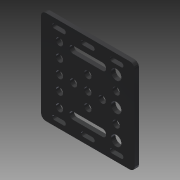
# Autodesk Inventor part: 20mm gantry plate
Saved by Autodesk Inventor 2014 SP1 (Build 180222100, 222)
## iProperties
Created: 2016-04-10
Part Number: 20mm gantry plate
Material: Generic
Document SubType Name: Modeling
Designer: Ben
Density: 1 g/cm^3
Appearance: Default
Author: Ben
Autodesk Inventor part; units mm, degrees
ref_plane "YZ Plane" through (0, 0, 0) normal (1, 0, 0) x (0, 1, 0)
ref_plane "XZ Plane" through (0, 0, 0) normal (0, 1, 0) x (-1, 0, 0)
ref_plane "XY Plane" through (0, 0, 0) normal (0, 0, 1) x (1, 0, 0)
sketch "Sketch1" plane through (0, 0, 0) normal (0, 0, 1) x (1, 0, 0)
  line L0 (-32.75, 32.75) -> (32.75, 32.75)
  line L1 (32.75, 32.75) -> (32.75, -32.75)
  line L2 (32.75, -32.75) -> (-32.75, -32.75)
  line L3 (-32.75, -32.75) -> (-32.75, 32.75)
  line L4 (0, 32.75) -> (0, -32.75) construction
  line L5 (-32.75, 0) -> (32.75, 0) construction
  point P0 (0, 0)
  dimension "d0" = 65.5
  dimension "d1" = 65.5
  constraints: 12 end point, 6 midpoint, 2 parallel, 1 horizontal, 1 perpendicular
  measures "d0" distance of L1.end L2.end
  measures "d1" distance of L0.end L1.end
extrude "Extrusion1" add sketch "Sketch1" along normal blind 3
sketch "Sketch2" plane through (0, 0, 3) normal (0, 0, 1) x (1, 0, 0)
  line L0 (32.75, 32.75) -> (-32.75, 32.75) projected
  line L1 (-32.75, 32.75) -> (-32.75, -32.75) projected
  line L2 (-32.75, -32.75) -> (32.75, -32.75) projected
  line L3 (32.75, -32.75) -> (32.75, 32.75) projected
  circle A0 centre (0, 0) radius 2.5
  circle A1 centre (0, 10) radius 2.5
  line L4 (0, 0) -> (0, 20.5611) construction
  circle A2 centre (-10, 0) radius 2.5
  circle A3 centre (0, -10) radius 2.5
  circle A4 centre (10, 0) radius 2.5
  circle A5 centre (-19.85, 0) radius 2.5
  circle A6 centre (-19.85, -10) radius 2.5
  circle A7 centre (-19.85, -20) radius 2.5
  circle A8 centre (-19.85, 10) radius 2.5
  circle A9 centre (-19.85, 0) radius 2.5
  circle A10 centre (-19.85, -10) radius 2.5
  circle A11 centre (-19.85, 20) radius 2.5
  circle A12 centre (-19.85, 10) radius 2.5
  circle A13 centre (-19.85, 0) radius 2.5
  line L5 (19.85, 32.75) -> (19.85, -32.75) construction
  circle A14 centre (19.85, 10) radius 2.5
  circle A15 centre (19.85, -10) radius 2.5
  line L6 (0, 0) -> (-32.75, 0) construction
  circle A16 centre (19.85, 0) radius 3.6
  circle A17 centre (19.85, 20) radius 3.6
  circle A18 centre (19.85, -20) radius 3.6
  circle A19 centre (19.85, 0) radius 3.6
  dimension "d4" = 5
  dimension "d5" = 5
  dimension "d6" = 10
  dimension "d9" = 360
  dimension "d11" = 5
  dimension "d12" = 12.9
  dimension "d15" = 10
  dimension "d18" = 10
  dimension "d21" = 5
  dimension "d22" = 5
  dimension "d23" = 12.9
  dimension "d24" = 10
  dimension "d25" = 7.2
  dimension "d28" = 20
  dimension "d31" = 20
  constraints: 20 centre point, 6 end point, 6 point on line, 4 vertical, 2 midpoint, 1 coincident, 1 parallel, 1 perpendicular, 1 symmetric about line, 31 other
  measures "d4" diameter of A0
  measures "d5" diameter of A1
  measures "d6" distance of L4.start A1.centre
  measures "d11" diameter of A5
  measures "d12" distance from line of A5.centre L1
  measures "d15" distance of A5.centre A6.centre
  measures "d18" distance of A5.centre A8.centre
  measures "d21" diameter of A14
  measures "d22" diameter of A15
  measures "d23" distance between parallel lines of L3 L5
  measures "d24" vertical distance of point (0, 0) A14.centre
  measures "d25" diameter of A16
  measures "d28" distance of A16.centre A17.centre
  measures "d31" distance of A16.centre A18.centre
extrude "Extrusion2" cut sketch "Sketch2" against normal up to next contours A0 | A1 | A2 | A3 | A4 | A5 | A6 | A7 | A8 | A11 | A14 | A15 | A16 | A17 | A18
sketch "Sketch3" plane through (0, 0, 3) normal (0, 0, 1) x (1, 0, 0)
  circle A0 centre (-19.85, -20) radius 2.5 projected
  circle A1 centre (0, 0) radius 2.5 projected
  line L0 (32.75, 32.75) -> (-32.75, 32.75) projected
  line L1 (-32.75, -32.75) -> (32.75, -32.75) projected
  line L2 (-10.32, -20) -> (10.32, -20) construction
  line L3 (-10.32, -22.5) -> (10.32, -22.5)
  line L4 (10.32, -17.5) -> (-10.32, -17.5)
  arc A2 (-10.32, -17.5) -> (-10.32, -22.5) centre (-10.32, -20) ccw
  arc A3 (10.32, -22.5) -> (10.32, -17.5) centre (10.32, -20) ccw
  line L5 (0, 0) -> (0, -39.6664) construction
  line L6 (0, 0) -> (-44.4767, 0) construction
  line L7 (-10.32, 20) -> (10.32, 20) construction
  line L8 (-10.32, 22.5) -> (10.32, 22.5)
  line L9 (10.32, 17.5) -> (-10.32, 17.5)
  arc A4 (-10.32, 22.5) -> (-10.32, 17.5) centre (-10.32, 20) ccw
  arc A5 (10.32, 17.5) -> (10.32, 22.5) centre (10.32, 20) ccw
  line L10 (-3.25, -27.7) -> (3.25, -27.7) construction
  line L11 (-3.25, -29.2) -> (3.25, -29.2)
  line L12 (3.25, -26.2) -> (-3.25, -26.2)
  arc A6 (-3.25, -26.2) -> (-3.25, -29.2) centre (-3.25, -27.7) ccw
  arc A7 (3.25, -29.2) -> (3.25, -26.2) centre (3.25, -27.7) ccw
  line L13 (16.9, -27.7) -> (23.4, -27.7) construction
  line L14 (16.9, -29.2) -> (23.4, -29.2)
  line L15 (23.4, -26.2) -> (16.9, -26.2)
  arc A8 (16.9, -26.2) -> (16.9, -29.2) centre (16.9, -27.7) ccw
  arc A9 (23.4, -29.2) -> (23.4, -26.2) centre (23.4, -27.7) ccw
  line L16 (-23.4, -27.7) -> (-16.9, -27.7) construction
  line L17 (-23.4, -29.2) -> (-16.9, -29.2)
  line L18 (-16.9, -26.2) -> (-23.4, -26.2)
  arc A10 (-23.4, -26.2) -> (-23.4, -29.2) centre (-23.4, -27.7) ccw
  arc A11 (-16.9, -29.2) -> (-16.9, -26.2) centre (-16.9, -27.7) ccw
  line L19 (-3.25, -27.7) -> (3.25, -27.7) construction
  line L20 (-3.25, -29.2) -> (3.25, -29.2)
  line L21 (3.25, -26.2) -> (-3.25, -26.2)
  arc A12 (-3.25, -26.2) -> (-3.25, -29.2) centre (-3.25, -27.7) ccw
  arc A13 (3.25, -29.2) -> (3.25, -26.2) centre (3.25, -27.7) ccw
  line L22 (-3.25, 27.7) -> (3.25, 27.7) construction
  line L23 (-3.25, 29.2) -> (3.25, 29.2)
  line L24 (3.25, 26.2) -> (-3.25, 26.2)
  arc A14 (-3.25, 29.2) -> (-3.25, 26.2) centre (-3.25, 27.7) ccw
  arc A15 (3.25, 26.2) -> (3.25, 29.2) centre (3.25, 27.7) ccw
  arc A16 (16.9, 29.2) -> (16.9, 26.2) centre (16.9, 27.7) ccw
  line L25 (23.4, 26.2) -> (16.9, 26.2)
  line L26 (16.9, 27.7) -> (23.4, 27.7) construction
  line L27 (16.9, 29.2) -> (23.4, 29.2)
  arc A17 (23.4, 26.2) -> (23.4, 29.2) centre (23.4, 27.7) ccw
  arc A18 (-23.4, 29.2) -> (-23.4, 26.2) centre (-23.4, 27.7) ccw
  line L28 (-16.9, 26.2) -> (-23.4, 26.2)
  line L29 (-23.4, 27.7) -> (-16.9, 27.7) construction
  line L30 (-23.4, 29.2) -> (-16.9, 29.2)
  arc A19 (-16.9, 26.2) -> (-16.9, 29.2) centre (-16.9, 27.7) ccw
  arc A20 (-3.25, 29.2) -> (-3.25, 26.2) centre (-3.25, 27.7) ccw
  line L31 (3.25, 26.2) -> (-3.25, 26.2)
  line L32 (-3.25, 27.7) -> (3.25, 27.7) construction
  line L33 (-3.25, 29.2) -> (3.25, 29.2)
  arc A21 (3.25, 26.2) -> (3.25, 29.2) centre (3.25, 27.7) ccw
  point P0 (0, -20)
  point P1 (0, 20)
  point P2 (0, -27.7)
  point P3 (20.15, -27.7)
  point P4 (-20.15, -27.7)
  point P5 (0, -27.7)
  point P6 (0, 27.7)
  point P7 (20.15, 27.7)
  point P8 (-20.15, 27.7)
  point P9 (0, 27.7)
  dimension "d36" = 5
  dimension "d37" = 20.64
  dimension "d38" = 3
  dimension "d39" = 60.45
  dimension "d40" = 6.5
  dimension "d43" = 20.15
  dimension "d46" = 20.15
  constraints: 84 end point, 40 point on circle, 35 symmetric about line, 20 centre point, 8 tangent, 4 parallel, 3 point on line, 2 horizontal, 2 midpoint, 2 perpendicular, 46 other
  measures "d36" diameter of A3
  measures "d37" distance of L2.end L2.start
  measures "d38" diameter of A7
  measures "d39" distance between parallel lines of L0 L10
  measures "d40" distance of L10.end L10.start
  measures "d43" distance of L12.end L15.end
  measures "d46" distance of L12.end L18.end
extrude "Extrusion3" cut sketch "Sketch3" against normal up to next contours A2 L4 A3 L3 | L8 A5 L9 A4 | A6 L12 A7 L11 | A8 L15 A9 L14 | A10 L18 A11 L17 | L23 A15 L24 A14 | L27 A17 L25 A16 | L30 A19 L28 A18
fillet "Fillet1" radius 3.38 4 edges at (32.75, -32.75, 1.5) (32.75, 32.75, 1.5) (-32.75, -32.75, 1.5) (-32.75, 32.75, 1.5)
body "Solid1"
